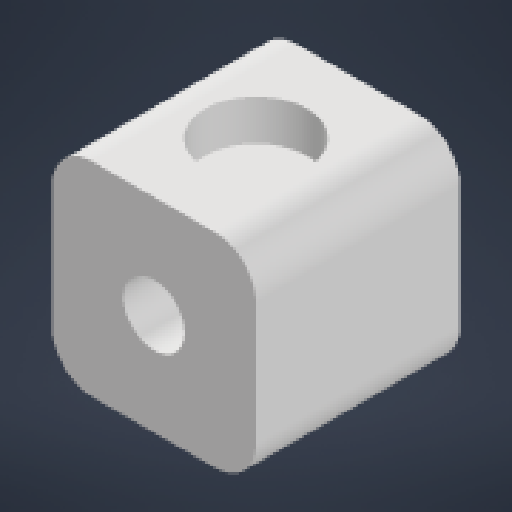
# Autodesk Inventor part: Claw Connector New
Saved by Autodesk Inventor 2023.6 (Build 276521000, 521)
## iProperties
Created: 2026-03-04
Part Number: Claw Connector New
Material: Generic
Document SubType Name: Modeling
Designer: user
Density: 1 g/cm^3
Appearance: Default
Author: user
Autodesk Inventor part; units mm, degrees
ref_plane "YZ Plane" through (0, 0, 0) normal (1, 0, 0) x (0, 1, 0)
ref_plane "XZ Plane" through (0, 0, 0) normal (0, 1, 0) x (-1, 0, 0)
ref_plane "XY Plane" through (0, 0, 0) normal (0, 0, 1) x (1, 0, 0)
sketch "Sketch1" plane through (0, 0, 0) normal (0, 0, 1) x (1, 0, 0)
  line L0 (-19.7239, 24.3858) -> (-9.7239, 24.3858)
  line L1 (-9.7239, 24.3858) -> (-9.7239, 14.3858)
  line L2 (-9.7239, 14.3858) -> (-19.7239, 14.3858)
  line L3 (-19.7239, 14.3858) -> (-19.7239, 24.3858)
  line L4 (-19.7239, 24.3858) -> (-9.7239, 14.3858) construction
  line L5 (-9.7239, 24.3858) -> (-19.7239, 14.3858) construction
  line L6 (-7.848, 12.2173) -> (-10.7345, 12.2561) projected
  line L7 (-7.848, 12.2173) -> (-12.5422, 20.6065) projected
  arc A0 (-12.5422, 20.6065) -> (-16.9056, 18.165) centre (-14.7239, 19.3858) ccw projected
  line L8 (-16.9056, 18.165) -> (-10.8018, 7.2566) projected
  line L9 (-10.7345, 12.2561) -> (-10.8018, 7.2566) projected
  circle A1 centre (-14.7239, 19.3858) radius 1.5 projected
  circle A2 centre (-14.7239, 19.3858) radius 1.5 projected
  line L10 (-68.8088, 12.3105) -> (-68.8088, 17.3105) projected
  arc A3 (-68.8088, 17.3105) -> (-78.8088, 17.3105) centre (-73.8088, 17.3105) ccw projected
  line L11 (-78.8088, 17.3105) -> (-78.8088, -37.6895) projected
  line L12 (-78.8088, -37.6895) -> (-33.8088, -37.6895) projected
  line L13 (-33.8088, -37.6895) -> (-28.8088, -32.6895) projected
  line L14 (-28.8088, -32.6895) -> (-73.8088, -32.6895) projected
  line L15 (-73.8088, -32.6895) -> (-73.8088, 7.3105) projected
  line L16 (-73.8088, 7.3105) -> (-18.8088, 7.3105) projected
  line L17 (-18.8088, 7.3105) -> (-12.5588, 18.1358) projected
  arc A4 (-12.5588, 18.1358) -> (-16.8889, 20.6358) centre (-14.7239, 19.3858) ccw projected
  line L18 (-16.8889, 20.6358) -> (-21.6956, 12.3105) projected
  line L19 (-21.6956, 12.3105) -> (-68.8088, 12.3105) projected
  circle A5 centre (-73.8088, 17.3105) radius 2.5 projected
  dimension "d0" = 10
  dimension "d1" = 10
  constraints: 12 end point, 2 parallel, 1 coincident, 1 horizontal, 1 midpoint, 1 perpendicular
  measures "d0" distance between parallel lines of L1 L3
  measures "d1" distance between parallel lines of L2 L0
extrude "Extrusion1" add sketch "Sketch1" along normal blind 13 contours L0 L1 L7 A0 L18 L3 | L18 A0 L8 L2 L3 | L1 L2 L17 A4 L7 | A0 A4 L17 L2 L8 | A1
fillet "Fillet1" radius 2 4 edges at (-9.7239, 24.3858, 6.5) (-9.7239, 14.3858, 6.5) (-19.7239, 24.3858, 6.5) (-19.7239, 14.3858, 6.5)
sketch "Sketch2" plane through (0, 0, 13) normal (0, 0, 1) x (1, 0, 0)
  circle A0 centre (-14.7239, 19.3858) radius 1.5 projected
  point P0 (0, 0)
extrude "Extrusion2" cut sketch "Sketch2" against normal blind 10
sketch "Sketch3" plane through (-17.7239, 24.3858, 0) normal (0, 1, 0) x (1, 0, 0)
  line L0 (0, -13) -> (0, 0) projected
  line L1 (6, -13) -> (0, -13) projected
  line L2 (6, 0) -> (6, -13) projected
  line L3 (6, 0) -> (0, 0) projected
  line L4 (0, -13) -> (0, 0) projected
  line L5 (0, -6.5) -> (6, -6.5)
  line L6 (6, 0) -> (6, -13) projected
  circle A0 centre (3, -6.5) radius 2.5
  point P0 (17.7239, 0)
  dimension "d7" = 5
  constraints: 3 midpoint, 2 end point, 1 centre point
  measures "d7" diameter of A0
extrude "Extrusion3" cut sketch "Sketch3" against normal blind 2 contours A0 L5 | L5 A0
body "Solid1"
